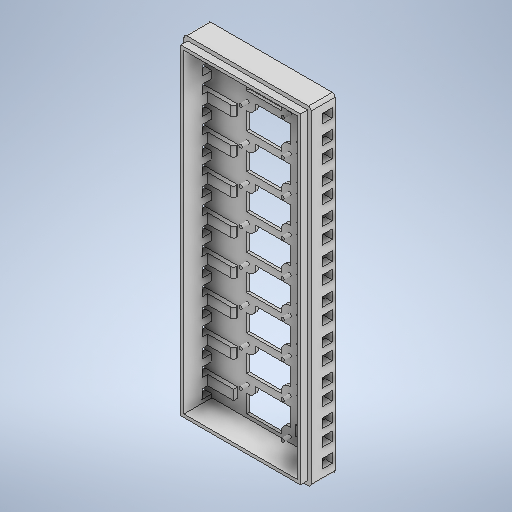
# Autodesk Inventor part: lm2596_socket_test
Saved by Autodesk Inventor 2025 (Build 290162000, 162)
## iProperties
Created: 2025-01-25
Part Number: lm2596_socket_test
Material: Všeobecné
Document SubType Name: Modeling
Designer: lukas
Density: 1 g/cm^3
Appearance: Výchozí
Author: lukas
## iProperties of the stored document lm2596_socket_3D tisk.ipt
Created: 2025-01-29
Part Number: lm2596_socket_3D tisk
Material: Všeobecné
Document SubType Name: Modeling
Designer: lukas
Density: 1 g/cm^3
Appearance: Výchozí
Author: lukas
Autodesk Inventor part; units mm, degrees
ref_plane "YZ Plane" through (0, 0, 0) normal (1, 0, 0) x (0, 1, 0)
ref_plane "XZ Plane" through (0, 0, 0) normal (0, 1, 0) x (-1, 0, 0)
sketch "Náčrt1" plane through (0, 0, 0) normal (0, 0, 1) x (1, 0, 0)
  line L0 (0, 17.5) -> (0, -17.5) projected
  line L1 (-32.9, 0) -> (32.9, 0) projected
  line L2 (23.5, -12.5) -> (-23.5, -12.5)
  line L3 (-23.5, -12.5) -> (-23.5, 12.5)
  line L4 (-23.5, 12.5) -> (23.5, 12.5)
  line L5 (23.5, 12.5) -> (23.5, -12.5)
  point P0 (0, 0)
  dimension "d0" = 47
  dimension "d1" = 25
  constraints: 8 end point, 2 parallel, 1 horizontal, 1 perpendicular, 2 other
  measures "d0" distance between parallel lines of L3 L5
  measures "d1" distance between parallel lines of L4 L2
extrude "Vysunutí1" add sketch "Náčrt1" along normal blind 2
sketch "Náčrt2" plane through (0, 0, 2) normal (0, 0, 1) x (1, 0, 0)
  line L0 (23.5, 12.5) -> (-23.5, 12.5) projected
  line L1 (-23.5, 12.5) -> (-23.5, -12.5) projected
  line L2 (-23.5, -12.5) -> (23.5, -12.5) projected
  line L3 (23.5, -12.5) -> (23.5, 12.5) projected
  line L4 (0, 17.5) -> (0, -17.5) projected
  line L5 (-32.9, 0) -> (32.9, 0) projected
  circle A0 centre (-15, 8.5) radius 1.2
  circle A1 centre (15, -8.5) radius 1.2
  point P0 (0, 0)
  dimension "d4" = 2.4
  dimension "d5" = 4
  dimension "d9" = 180
  dimension "d18" = 8.5
  constraints: 2 centre point, 3 other
  measures "d4" diameter of A0
  measures "d5" distance from line of A0.centre L0
  measures "d18" distance from line of L1 A0.centre
extrude "Vysunutí2" add sketch "Náčrt2" along normal blind 5 contours A0 | A1
sketch "Náčrt3" plane through (0, 0, 2) normal (0, 0, 1) x (1, 0, 0)
  circle A0 centre (15, -8.5) radius 1.2 projected
  circle A1 centre (-15, 8.5) radius 1.2 projected
  line L0 (23.5, 12.5) -> (-23.5, 12.5) projected
  line L1 (-23.5, 12.5) -> (-23.5, -12.5) projected
  line L2 (-23.5, -12.5) -> (23.5, -12.5) projected
  line L3 (23.5, -12.5) -> (23.5, 12.5) projected
  line L4 (0, 17.5) -> (0, -17.5) projected
  line L5 (-32.9, 0) -> (32.9, 0) projected
  line L6 (-23.5, 12.5) -> (-23.5, -12.5) projected
  line L7 (-22, -3.5) -> (-23.5, -3.5)
  line L8 (-23.5, -3.5) -> (-23.5, 3.5)
  line L9 (-23.5, 3.5) -> (-22, 3.5)
  line L10 (-22, 3.5) -> (-22, -3.5)
  line L11 (23.5, -3.5) -> (22, -3.5)
  line L12 (22, -3.5) -> (22, 3.5)
  line L13 (22, 3.5) -> (23.5, 3.5)
  line L14 (23.5, 3.5) -> (23.5, -3.5)
  line L15 (22, -3.5) -> (23.5, -3.5)
  line L16 (23.5, -3.5) -> (23.5, 0)
  line L17 (23.5, 0) -> (22, 0)
  line L18 (22, 0) -> (22, -3.5)
  line L19 (-22, -3.5) -> (-23.5, -3.5)
  line L20 (-23.5, -3.5) -> (-23.5, 0)
  line L21 (-23.5, 0) -> (-22, 0)
  line L22 (-22, 0) -> (-22, -3.5)
  point P0 (0, 0)
  point P1 (22, 0)
  point P2 (-22, 0)
  point P3 (-23.5, 3.5)
  point P4 (-23.5, -3.5)
  dimension "d13" = 7
  dimension "d14" = 7
  dimension "d15" = 44
  constraints: 32 end point, 8 parallel, 4 horizontal, 4 perpendicular, 2 midpoint, 2 point on line, 3 other
  measures "d13" distance of L9.end L7.start
  measures "d14" distance of L11.end L12.end
  measures "d15" distance between parallel lines of L10 L12
extrude "Vysunutí3" add sketch "Náčrt3" along normal blind 3 contours L3 L5 L12 L13 | L3 L11 L12 L5 | L9 L10 L5 L1 | L10 L7 L1 L5
sketch "Náčrt4" plane through (0, 0, 2) normal (0, 0, 1) x (1, 0, 0)
  line L0 (22, 3.5) -> (23.5, 3.5) projected
  line L1 (23.5, 3.5) -> (23.5, 12.5) projected
  line L2 (23.5, 12.5) -> (-23.5, 12.5) projected
  line L3 (-23.5, 12.5) -> (-23.5, 3.5) projected
  line L4 (-23.5, 3.5) -> (-22, 3.5) projected
  line L5 (-22, 3.5) -> (-22, -3.5) projected
  line L6 (-22, -3.5) -> (-23.5, -3.5) projected
  line L7 (-23.5, -3.5) -> (-23.5, -12.5) projected
  line L8 (-23.5, -12.5) -> (23.5, -12.5) projected
  line L9 (23.5, -12.5) -> (23.5, -3.5) projected
  line L10 (23.5, -3.5) -> (22, -3.5) projected
  line L11 (22, -3.5) -> (22, 3.5) projected
  circle A0 centre (15, -8.5) radius 1.2 projected
  circle A1 centre (-15, 8.5) radius 1.2 projected
  line L12 (15.8095, 10) -> (15.8095, -2.5549)
  line L13 (-15.8095, -10) -> (-15.8095, 2.5549)
  line L14 (0, 17.5) -> (0, -17.5) projected
  line L15 (-32.9, 0) -> (32.9, 0) projected
  arc A2 (-15.8095, 2.5549) -> (-9.1905, 10) centre (-15, 8.5) ccw
  arc A3 (15.8095, -2.5549) -> (9.1905, -10) centre (15, -8.5) ccw
  line L16 (-9.1905, 10) -> (15.8095, 10)
  line L17 (9.1905, -10) -> (-15.8095, -10)
  point P0 (0, 0)
  dimension "d21" = 12
  dimension "d22" = 12
  dimension "d23" = 20
  dimension "d25" = 25
  dimension "d26" = 25
  constraints: 8 end point, 4 point on circle, 2 centre point, 2 coincident, 2 parallel, 1 horizontal, 1 perpendicular, 1 other
  measures "d21" diameter of A2
  measures "d22" diameter of A3
  measures "d23" distance between parallel lines of L16 L17
  measures "d25" distance of L16.start L12.start
  measures "d26" distance of L17.start L13.start
extrude "Vysunutí4" cut sketch "Náčrt4" against normal through all contours L15 L14 L16 L12 | L12 A3 L17 L14 L15 | L15 L13 A2 L16 L14 | L14 L17 L13 L15
pattern_linear "Obdélníkové pole1" count 9 spacing 25 along (0, 1, 0) first direction both ways yes
sketch "Náčrt12" plane through (0, 0, 0) normal (0, 0, -1) x (-1, 0, 0)
  line L0 (15.8095, 15) -> (-9.1905, 15) projected
  arc A0 (-9.1905, 15) -> (-15.8095, 22.4451) centre (-15, 16.5) ccw projected
  line L1 (-15.8095, 22.4451) -> (-15.8095, 35) projected
  line L2 (-15.8095, 35) -> (9.1905, 35) projected
  arc A1 (9.1905, 35) -> (15.8095, 27.5549) centre (15, 33.5) ccw projected
  line L3 (15.8095, 27.5549) -> (15.8095, 15) projected
  line L4 (15.8095, 40) -> (-9.1905, 40) projected
  arc A2 (-9.1905, 40) -> (-15.8095, 47.4451) centre (-15, 41.5) ccw projected
  line L5 (-15.8095, 47.4451) -> (-15.8095, 60) projected
  line L6 (-15.8095, 60) -> (9.1905, 60) projected
  arc A3 (9.1905, 60) -> (15.8095, 52.5549) centre (15, 58.5) ccw projected
  line L7 (15.8095, 52.5549) -> (15.8095, 40) projected
  line L8 (15.8095, 65) -> (-9.1905, 65) projected
  arc A4 (-9.1905, 65) -> (-15.8095, 72.4451) centre (-15, 66.5) ccw projected
  line L9 (-15.8095, 72.4451) -> (-15.8095, 85) projected
  line L10 (-15.8095, 85) -> (9.1905, 85) projected
  arc A5 (9.1905, 85) -> (15.8095, 77.5549) centre (15, 83.5) ccw projected
  line L11 (15.8095, 77.5549) -> (15.8095, 65) projected
  line L12 (15.8095, 90) -> (-9.1905, 90) projected
  arc A6 (-9.1905, 90) -> (-15.8095, 97.4451) centre (-15, 91.5) ccw projected
  line L13 (-15.8095, 97.4451) -> (-15.8095, 110) projected
  line L14 (-15.8095, 110) -> (9.1905, 110) projected
  arc A7 (9.1905, 110) -> (15.8095, 102.5549) centre (15, 108.5) ccw projected
  line L15 (15.8095, 102.5549) -> (15.8095, 90) projected
  line L16 (15.8095, -110) -> (-9.1905, -110) projected
  arc A8 (-9.1905, -110) -> (-15.8095, -102.5549) centre (-15, -108.5) ccw projected
  line L17 (-15.8095, -102.5549) -> (-15.8095, -90) projected
  line L18 (-15.8095, -90) -> (9.1905, -90) projected
  arc A9 (9.1905, -90) -> (15.8095, -97.4451) centre (15, -91.5) ccw projected
  line L19 (15.8095, -97.4451) -> (15.8095, -110) projected
  line L20 (15.8095, -85) -> (-9.1905, -85) projected
  arc A10 (-9.1905, -85) -> (-15.8095, -77.5549) centre (-15, -83.5) ccw projected
  line L21 (-15.8095, -77.5549) -> (-15.8095, -65) projected
  line L22 (-15.8095, -65) -> (9.1905, -65) projected
  arc A11 (9.1905, -65) -> (15.8095, -72.4451) centre (15, -66.5) ccw projected
  line L23 (15.8095, -72.4451) -> (15.8095, -85) projected
  line L24 (15.8095, -60) -> (-9.1905, -60) projected
  arc A12 (-9.1905, -60) -> (-15.8095, -52.5549) centre (-15, -58.5) ccw projected
  line L25 (-15.8095, -52.5549) -> (-15.8095, -40) projected
  line L26 (-15.8095, -40) -> (9.1905, -40) projected
  arc A13 (9.1905, -40) -> (15.8095, -47.4451) centre (15, -41.5) ccw projected
  line L27 (15.8095, -47.4451) -> (15.8095, -60) projected
  line L28 (15.8095, -35) -> (-9.1905, -35) projected
  arc A14 (-9.1905, -35) -> (-15.8095, -27.5549) centre (-15, -33.5) ccw projected
  line L29 (-15.8095, -27.5549) -> (-15.8095, -15) projected
  line L30 (-15.8095, -15) -> (9.1905, -15) projected
  arc A15 (9.1905, -15) -> (15.8095, -22.4451) centre (15, -16.5) ccw projected
  line L31 (15.8095, -22.4451) -> (15.8095, -35) projected
  line L32 (15.8095, -10) -> (-9.1905, -10) projected
  arc A16 (-9.1905, -10) -> (-15.8095, -2.5549) centre (-15, -8.5) ccw projected
  line L33 (-15.8095, -2.5549) -> (-15.8095, 10) projected
  line L34 (-15.8095, 10) -> (9.1905, 10) projected
  arc A17 (9.1905, 10) -> (15.8095, 2.5549) centre (15, 8.5) ccw projected
  line L35 (15.8095, 2.5549) -> (15.8095, -10) projected
  line L36 (-23.5, -112.5) -> (-23.5, 112.5) projected
  line L37 (23.5, -112.5) -> (-23.5, -112.5) projected
  line L38 (23.5, 112.5) -> (23.5, -112.5) projected
  line L39 (-23.5, 112.5) -> (23.5, 112.5) projected
  line L40 (-45.5, 117.5) -> (45.5, 117.5)
  line L41 (45.5, 117.5) -> (45.5, -117.5)
  line L42 (45.5, -117.5) -> (-45.5, -117.5)
  line L43 (-45.5, -117.5) -> (-45.5, 117.5)
  line L44 (0, -164.5) -> (0, 164.5) projected
  line L45 (-63.7, 0) -> (63.7, 0) projected
  point P0 (0, 0)
  dimension "d53" = 22
  dimension "d54" = 5
  constraints: 8 end point, 2 parallel, 1 horizontal, 1 perpendicular, 2 other
  measures "d53" distance between parallel lines of L43 L36
  measures "d54" distance between parallel lines of L37 L42
extrude "Vysunutí12" add sketch "Náčrt12" against normal blind 2 contours L45 L43 L40 L44 L39 L36 | L36 L37 L44 L42 L43 L45 | L45 L41 L42 L44 L37 L38 | L38 L39 L44 L40 L41 L45
sketch "Náčrt13" plane through (0, 0, 2) normal (0, 0, 1) x (1, 0, 0)
  line L0 (-23.5, -21.5) -> (-22, -21.5) projected
  line L1 (-22, -21.5) -> (-22, -28.5) projected
  line L2 (-22, -28.5) -> (-23.5, -28.5) projected
  line L3 (-23.5, -21.5) -> (-23.5, -28.5) projected
  line L4 (-23.5, -46.5) -> (-22, -46.5) projected
  line L5 (-22, -46.5) -> (-22, -53.5) projected
  line L6 (-22, -53.5) -> (-23.5, -53.5) projected
  line L7 (-23.5, -46.5) -> (-23.5, -53.5) projected
  line L8 (-23.5, 3.5) -> (-23.5, -3.5) projected
  line L9 (-23.5, 3.5) -> (-22, 3.5) projected
  line L10 (-22, 3.5) -> (-22, -3.5) projected
  line L11 (-22, -3.5) -> (-23.5, -3.5) projected
  line L12 (-23.5, -71.5) -> (-22, -71.5) projected
  line L13 (-22, -71.5) -> (-22, -78.5) projected
  line L14 (-22, -78.5) -> (-23.5, -78.5) projected
  line L15 (-23.5, -71.5) -> (-23.5, -78.5) projected
  line L16 (23.5, -28.5) -> (22, -28.5) projected
  line L17 (22, -28.5) -> (22, -21.5) projected
  line L18 (22, -21.5) -> (23.5, -21.5) projected
  line L19 (23.5, -28.5) -> (23.5, -21.5) projected
  line L20 (23.5, -53.5) -> (23.5, -46.5) projected
  line L21 (23.5, -53.5) -> (22, -53.5) projected
  line L22 (22, -53.5) -> (22, -46.5) projected
  line L23 (22, -46.5) -> (23.5, -46.5) projected
  line L24 (-23.5, 28.5) -> (-23.5, 21.5) projected
  line L25 (-23.5, 28.5) -> (-22, 28.5) projected
  line L26 (-22, 28.5) -> (-22, 21.5) projected
  line L27 (-22, 21.5) -> (-23.5, 21.5) projected
  line L28 (-23.5, -96.5) -> (-22, -96.5) projected
  line L29 (-22, -96.5) -> (-22, -103.5) projected
  line L30 (-22, -103.5) -> (-23.5, -103.5) projected
  line L31 (-23.5, -96.5) -> (-23.5, -103.5) projected
  line L32 (23.5, -3.5) -> (22, -3.5) projected
  line L33 (22, -3.5) -> (22, 3.5) projected
  line L34 (22, 3.5) -> (23.5, 3.5) projected
  line L35 (23.5, -3.5) -> (23.5, 3.5) projected
  line L36 (23.5, -78.5) -> (23.5, -71.5) projected
  line L37 (23.5, -78.5) -> (22, -78.5) projected
  line L38 (22, -78.5) -> (22, -71.5) projected
  line L39 (22, -71.5) -> (23.5, -71.5) projected
  line L40 (-23.5, 53.5) -> (-23.5, 46.5) projected
  line L41 (-23.5, 53.5) -> (-22, 53.5) projected
  line L42 (-22, 53.5) -> (-22, 46.5) projected
  line L43 (-22, 46.5) -> (-23.5, 46.5) projected
  line L44 (23.5, 21.5) -> (22, 21.5) projected
  line L45 (22, 21.5) -> (22, 28.5) projected
  line L46 (22, 28.5) -> (23.5, 28.5) projected
  line L47 (23.5, 21.5) -> (23.5, 28.5) projected
  line L48 (23.5, -103.5) -> (23.5, -96.5) projected
  line L49 (23.5, -103.5) -> (22, -103.5) projected
  line L50 (22, -103.5) -> (22, -96.5) projected
  line L51 (22, -96.5) -> (23.5, -96.5) projected
  line L52 (-23.5, 78.5) -> (-23.5, 71.5) projected
  line L53 (-23.5, 78.5) -> (-22, 78.5) projected
  line L54 (-22, 78.5) -> (-22, 71.5) projected
  line L55 (-22, 71.5) -> (-23.5, 71.5) projected
  line L56 (23.5, 46.5) -> (22, 46.5) projected
  line L57 (22, 46.5) -> (22, 53.5) projected
  line L58 (22, 53.5) -> (23.5, 53.5) projected
  line L59 (23.5, 46.5) -> (23.5, 53.5) projected
  line L60 (23.5, 71.5) -> (22, 71.5) projected
  line L61 (22, 71.5) -> (22, 78.5) projected
  line L62 (22, 78.5) -> (23.5, 78.5) projected
  line L63 (23.5, 71.5) -> (23.5, 78.5) projected
  line L64 (-23.5, 103.5) -> (-23.5, 96.5) projected
  line L65 (-23.5, 103.5) -> (-22, 103.5) projected
  line L66 (-22, 103.5) -> (-22, 96.5) projected
  line L67 (-22, 96.5) -> (-23.5, 96.5) projected
  line L68 (45.5, -117.5) -> (45.5, 117.5) projected
  line L69 (45.5, 117.5) -> (-45.5, 117.5) projected
  line L70 (-45.5, 117.5) -> (-45.5, -117.5) projected
  line L71 (-45.5, -117.5) -> (45.5, -117.5) projected
  circle A0 centre (-15, 33.5) radius 1.2 projected
  circle A1 centre (15, 16.5) radius 1.2 projected
  line L72 (9.1905, 15) -> (-15.8095, 15) projected
  line L73 (-15.8095, 15) -> (-15.8095, 27.5549) projected
  arc A2 (-15.8095, 27.5549) -> (-9.1905, 35) centre (-15, 33.5) ccw projected
  line L74 (-9.1905, 35) -> (15.8095, 35) projected
  line L75 (15.8095, 35) -> (15.8095, 22.4451) projected
  arc A3 (15.8095, 22.4451) -> (9.1905, 15) centre (15, 16.5) ccw projected
  line L76 (9.1905, 40) -> (-15.8095, 40) projected
  line L77 (-15.8095, 40) -> (-15.8095, 52.5549) projected
  arc A4 (-15.8095, 52.5549) -> (-9.1905, 60) centre (-15, 58.5) ccw projected
  line L78 (-9.1905, 60) -> (15.8095, 60) projected
  line L79 (15.8095, 60) -> (15.8095, 47.4451) projected
  arc A5 (15.8095, 47.4451) -> (9.1905, 40) centre (15, 41.5) ccw projected
  circle A6 centre (15, 41.5) radius 1.2 projected
  circle A7 centre (-15, 58.5) radius 1.2 projected
  line L80 (9.1905, 65) -> (-15.8095, 65) projected
  line L81 (-15.8095, 65) -> (-15.8095, 77.5549) projected
  arc A8 (-15.8095, 77.5549) -> (-9.1905, 85) centre (-15, 83.5) ccw projected
  line L82 (-9.1905, 85) -> (15.8095, 85) projected
  line L83 (15.8095, 85) -> (15.8095, 72.4451) projected
  arc A9 (15.8095, 72.4451) -> (9.1905, 65) centre (15, 66.5) ccw projected
  circle A10 centre (15, 66.5) radius 1.2 projected
  circle A11 centre (-15, 83.5) radius 1.2 projected
  line L84 (9.1905, 90) -> (-15.8095, 90) projected
  line L85 (-15.8095, 90) -> (-15.8095, 102.5549) projected
  arc A12 (-15.8095, 102.5549) -> (-9.1905, 110) centre (-15, 108.5) ccw projected
  line L86 (-9.1905, 110) -> (15.8095, 110) projected
  line L87 (15.8095, 110) -> (15.8095, 97.4451) projected
  arc A13 (15.8095, 97.4451) -> (9.1905, 90) centre (15, 91.5) ccw projected
  circle A14 centre (15, 91.5) radius 1.2 projected
  circle A15 centre (-15, 108.5) radius 1.2 projected
  circle A16 centre (-15, -91.5) radius 1.2 projected
  circle A17 centre (15, -108.5) radius 1.2 projected
  line L88 (9.1905, -110) -> (-15.8095, -110) projected
  line L89 (-15.8095, -110) -> (-15.8095, -97.4451) projected
  arc A18 (-15.8095, -97.4451) -> (-9.1905, -90) centre (-15, -91.5) ccw projected
  line L90 (-9.1905, -90) -> (15.8095, -90) projected
  line L91 (15.8095, -90) -> (15.8095, -102.5549) projected
  arc A19 (15.8095, -102.5549) -> (9.1905, -110) centre (15, -108.5) ccw projected
  line L92 (9.1905, -85) -> (-15.8095, -85) projected
  line L93 (-15.8095, -85) -> (-15.8095, -72.4451) projected
  arc A20 (-15.8095, -72.4451) -> (-9.1905, -65) centre (-15, -66.5) ccw projected
  line L94 (-9.1905, -65) -> (15.8095, -65) projected
  line L95 (15.8095, -65) -> (15.8095, -77.5549) projected
  arc A21 (15.8095, -77.5549) -> (9.1905, -85) centre (15, -83.5) ccw projected
  circle A22 centre (15, -83.5) radius 1.2 projected
  circle A23 centre (-15, -66.5) radius 1.2 projected
  line L96 (9.1905, -60) -> (-15.8095, -60) projected
  line L97 (-15.8095, -60) -> (-15.8095, -47.4451) projected
  arc A24 (-15.8095, -47.4451) -> (-9.1905, -40) centre (-15, -41.5) ccw projected
  line L98 (-9.1905, -40) -> (15.8095, -40) projected
  line L99 (15.8095, -40) -> (15.8095, -52.5549) projected
  arc A25 (15.8095, -52.5549) -> (9.1905, -60) centre (15, -58.5) ccw projected
  circle A26 centre (15, -58.5) radius 1.2 projected
  circle A27 centre (-15, -41.5) radius 1.2 projected
  line L100 (9.1905, -35) -> (-15.8095, -35) projected
  line L101 (-15.8095, -35) -> (-15.8095, -22.4451) projected
  arc A28 (-15.8095, -22.4451) -> (-9.1905, -15) centre (-15, -16.5) ccw projected
  line L102 (-9.1905, -15) -> (15.8095, -15) projected
  line L103 (15.8095, -15) -> (15.8095, -27.5549) projected
  arc A29 (15.8095, -27.5549) -> (9.1905, -35) centre (15, -33.5) ccw projected
  circle A30 centre (15, -33.5) radius 1.2 projected
  circle A31 centre (-15, -16.5) radius 1.2 projected
  line L104 (9.1905, -10) -> (-15.8095, -10) projected
  line L105 (-15.8095, -10) -> (-15.8095, 2.5549) projected
  arc A32 (-15.8095, 2.5549) -> (-9.1905, 10) centre (-15, 8.5) ccw projected
  line L106 (-9.1905, 10) -> (15.8095, 10) projected
  line L107 (15.8095, 10) -> (15.8095, -2.5549) projected
  arc A33 (15.8095, -2.5549) -> (9.1905, -10) centre (15, -8.5) ccw projected
  line L108 (23.5, 96.5) -> (23.5, 103.5) projected
  line L109 (23.5, 96.5) -> (22, 96.5) projected
  line L110 (22, 96.5) -> (22, 103.5) projected
  line L111 (22, 103.5) -> (23.5, 103.5) projected
  circle A34 centre (15, -8.5) radius 1.2 projected
  circle A35 centre (-15, 8.5) radius 1.2 projected
  line L112 (0, 164.5) -> (0, -164.5) projected
  line L113 (-63.7, 0) -> (63.7, 0) projected
  line L114 (45.5, -117.5) -> (45.5, 117.5) projected
  line L115 (45.5, 117.5) -> (-45.5, 117.5)
  line L116 (-45.5, 117.5) -> (-45.5, -117.5)
  line L117 (-45.5, -117.5) -> (45.5, -117.5)
  line L118 (45.5, -117.5) -> (45.5, 117.5)
  line L119 (40.5, 112.5) -> (-40.5, 112.5)
  line L120 (-40.5, 112.5) -> (-40.5, -112.5)
  line L121 (-40.5, -112.5) -> (40.5, -112.5)
  line L122 (40.5, -112.5) -> (40.5, 112.5)
  line L123 (45.5, 117.5) -> (-45.5, 117.5)
  line L124 (-45.5, 117.5) -> (-45.5, -117.5)
  line L125 (-45.5, -117.5) -> (45.5, -117.5)
  line L126 (45.5, -117.5) -> (45.5, 117.5)
  line L127 (45.5, 0) -> (40.5, 0)
  line L128 (40.5, -112.5) -> (0, -112.5)
  line L129 (-40.5, -112.5) -> (-40.5, 0)
  line L130 (-45.5, 117.5) -> (-45.5, -117.5) projected
  line L131 (-45.5, 0) -> (-45.5, -117.5)
  line L132 (-45.5, -117.5) -> (45.5, -117.5)
  line L133 (45.5, 0) -> (45.5, -117.5)
  line L134 (40.5, 0) -> (40.5, -112.5)
  line L135 (0, -112.5) -> (40.5, -112.5)
  line L136 (-45.5, -117.5) -> (45.5, -117.5) projected
  line L137 (0, -117.5) -> (0, -112.5)
  line L138 (0, -117.5) -> (45.5, -117.5)
  line L139 (45.5, -117.5) -> (45.5, 0)
  line L140 (45.5, 0) -> (40.5, 0)
  point P0 (0, 0)
  dimension "d59" = 5
  constraints: 48 end point, 6 midpoint, 6 parallel, 6 perpendicular, 5 collinear, 2 horizontal, 1 vertical, 3 other
  measures "d59" distance between parallel lines of L118 L122
extrude "Vysunutí13" add sketch "Náčrt13" along normal blind 15 contours L120 L121 L112 L71 L70 L113 | L113 L70 L69 L112 L119 L120 | L112 L69 L68 L113 L122 L119 | L121 L122 L113 L68 L71 L112
sketch "Náčrt14" plane through (-45.5, -117.5, 0) normal (-1, 0, 0) x (0, 0, 1)
  line L0 (-3.4, 117.5) -> (20.4, 117.5) projected
  line L1 (0, 282) -> (0, -47) projected
  line L2 (2, 230) -> (17, 230) projected
  line L3 (2, 230) -> (17, 230) projected
  line L4 (2, 221) -> (2, 214) projected
  line L5 (2, 214) -> (5, 214) projected
  line L6 (5, 221) -> (5, 214) projected
  line L7 (2, 221) -> (5, 221) projected
  line L8 (2, 5) -> (2, 230) projected
  line L9 (2, 230) -> (2, 5) projected
  line L10 (2, 96) -> (2, 89) projected
  line L11 (2, 96) -> (2, 89) projected
  line L12 (2, 71) -> (2, 64) projected
  line L13 (2, 71) -> (2, 64) projected
  line L14 (2, 121) -> (2, 114) projected
  line L15 (2, 121) -> (2, 114) projected
  line L16 (2, 46) -> (2, 39) projected
  line L17 (2, 46) -> (2, 39) projected
  line L18 (2, 89) -> (2, 96) projected
  line L19 (2, 89) -> (2, 96) projected
  line L20 (2, 64) -> (2, 71) projected
  line L21 (2, 64) -> (2, 71) projected
  line L22 (2, 146) -> (2, 139) projected
  line L23 (2, 146) -> (2, 139) projected
  line L24 (2, 21) -> (2, 14) projected
  line L25 (2, 21) -> (2, 14) projected
  line L26 (2, 114) -> (2, 121) projected
  line L27 (2, 114) -> (2, 121) projected
  line L28 (2, 39) -> (2, 46) projected
  line L29 (2, 39) -> (2, 46) projected
  line L30 (2, 171) -> (2, 164) projected
  line L31 (2, 171) -> (2, 164) projected
  line L32 (2, 139) -> (2, 146) projected
  line L33 (2, 139) -> (2, 146) projected
  line L34 (2, 14) -> (2, 21) projected
  line L35 (2, 14) -> (2, 21) projected
  line L36 (2, 196) -> (2, 189) projected
  line L37 (2, 196) -> (2, 189) projected
  line L38 (2, 164) -> (2, 171) projected
  line L39 (2, 164) -> (2, 171) projected
  line L40 (2, 189) -> (2, 196) projected
  line L41 (2, 189) -> (2, 196) projected
  line L42 (2, 221) -> (2, 214) projected
  line L43 (2, 221) -> (2, 214) projected
  line L44 (2, 152.2) -> (2, 149.8) projected
  line L45 (2, 135.2) -> (2, 132.8) projected
  line L46 (2, 132.5) -> (2, 145.0549) projected
  line L47 (2, 145.0549) -> (2, 152.5) projected
  line L48 (2, 152.5) -> (2, 139.9451) projected
  line L49 (2, 139.9451) -> (2, 132.5) projected
  line L50 (2, 157.5) -> (2, 170.0549) projected
  line L51 (2, 170.0549) -> (2, 177.5) projected
  line L52 (2, 177.5) -> (2, 164.9451) projected
  line L53 (2, 164.9451) -> (2, 157.5) projected
  line L54 (2, 160.2) -> (2, 157.8) projected
  line L55 (2, 177.2) -> (2, 174.8) projected
  line L56 (2, 182.5) -> (2, 195.0549) projected
  line L57 (2, 195.0549) -> (2, 202.5) projected
  line L58 (2, 202.5) -> (2, 189.9451) projected
  line L59 (2, 189.9451) -> (2, 182.5) projected
  line L60 (2, 185.2) -> (2, 182.8) projected
  line L61 (2, 202.2) -> (2, 199.8) projected
  line L62 (2, 207.5) -> (2, 220.0549) projected
  line L63 (2, 220.0549) -> (2, 227.5) projected
  line L64 (2, 227.5) -> (2, 214.9451) projected
  line L65 (2, 214.9451) -> (2, 207.5) projected
  line L66 (2, 210.2) -> (2, 207.8) projected
  line L67 (2, 227.2) -> (2, 224.8) projected
  line L68 (2, 27.2) -> (2, 24.8) projected
  line L69 (2, 10.2) -> (2, 7.8) projected
  line L70 (2, 7.5) -> (2, 20.0549) projected
  line L71 (2, 20.0549) -> (2, 27.5) projected
  line L72 (2, 27.5) -> (2, 14.9451) projected
  line L73 (2, 14.9451) -> (2, 7.5) projected
  line L74 (2, 32.5) -> (2, 45.0549) projected
  line L75 (2, 45.0549) -> (2, 52.5) projected
  line L76 (2, 52.5) -> (2, 39.9451) projected
  line L77 (2, 39.9451) -> (2, 32.5) projected
  line L78 (2, 35.2) -> (2, 32.8) projected
  line L79 (2, 52.2) -> (2, 49.8) projected
  line L80 (2, 57.5) -> (2, 70.0549) projected
  line L81 (2, 70.0549) -> (2, 77.5) projected
  line L82 (2, 77.5) -> (2, 64.9451) projected
  line L83 (2, 64.9451) -> (2, 57.5) projected
  line L84 (2, 60.2) -> (2, 57.8) projected
  line L85 (2, 77.2) -> (2, 74.8) projected
  line L86 (2, 82.5) -> (2, 95.0549) projected
  line L87 (2, 95.0549) -> (2, 102.5) projected
  line L88 (2, 102.5) -> (2, 89.9451) projected
  line L89 (2, 89.9451) -> (2, 82.5) projected
  line L90 (2, 85.2) -> (2, 82.8) projected
  line L91 (2, 102.2) -> (2, 99.8) projected
  line L92 (2, 107.5) -> (2, 120.0549) projected
  line L93 (2, 120.0549) -> (2, 127.5) projected
  line L94 (2, 127.5) -> (2, 114.9451) projected
  line L95 (2, 114.9451) -> (2, 107.5) projected
  line L96 (2, 214) -> (2, 221) projected
  line L97 (2, 214) -> (2, 221) projected
  line L98 (2, 110.2) -> (2, 107.8) projected
  line L99 (2, 127.2) -> (2, 124.8) projected
  line L100 (2, 5) -> (17, 5) projected
  line L101 (2, 230) -> (9, 230)
  line L102 (9, 230) -> (9, 5)
  line L103 (9, 5) -> (2, 5)
  line L104 (2, 5) -> (2, 230)
  line L105 (2, 196) -> (2, 189) projected
  line L106 (2, 189) -> (5, 189) projected
  line L107 (5, 196) -> (5, 189) projected
  line L108 (2, 196) -> (5, 196) projected
  line L109 (2, 171) -> (2, 164) projected
  line L110 (2, 164) -> (5, 164) projected
  line L111 (5, 171) -> (5, 164) projected
  line L112 (2, 171) -> (5, 171) projected
  line L113 (2, 146) -> (2, 139) projected
  line L114 (2, 139) -> (5, 139) projected
  line L115 (5, 146) -> (5, 139) projected
  line L116 (2, 146) -> (5, 146) projected
  line L117 (2, 121) -> (2, 114) projected
  line L118 (2, 114) -> (5, 114) projected
  line L119 (5, 121) -> (5, 114) projected
  line L120 (2, 121) -> (5, 121) projected
  line L121 (2, 96) -> (2, 89) projected
  line L122 (2, 89) -> (5, 89) projected
  line L123 (5, 96) -> (5, 89) projected
  line L124 (2, 96) -> (5, 96) projected
  line L125 (2, 71) -> (2, 64) projected
  line L126 (2, 64) -> (5, 64) projected
  line L127 (5, 71) -> (5, 64) projected
  line L128 (2, 71) -> (5, 71) projected
  line L129 (2, 46) -> (2, 39) projected
  line L130 (2, 39) -> (5, 39) projected
  line L131 (5, 46) -> (5, 39) projected
  line L132 (2, 46) -> (5, 46) projected
  line L133 (2, 21) -> (2, 14) projected
  line L134 (2, 14) -> (5, 14) projected
  line L135 (5, 21) -> (5, 14) projected
  line L136 (2, 21) -> (5, 21) projected
  line L137 (2, 221) -> (9, 221)
  line L138 (9, 221) -> (9, 214)
  line L139 (9, 214) -> (2, 214)
  line L140 (2, 214) -> (2, 221)
  line L141 (2, 196) -> (9, 196)
  line L142 (9, 196) -> (9, 189)
  line L143 (9, 189) -> (2, 189)
  line L144 (2, 189) -> (2, 196)
  line L145 (2, 171) -> (9, 171)
  line L146 (9, 171) -> (9, 164)
  line L147 (9, 164) -> (2, 164)
  line L148 (2, 164) -> (2, 171)
  line L149 (2, 146) -> (9, 146)
  line L150 (9, 146) -> (9, 139)
  line L151 (9, 139) -> (2, 139)
  line L152 (2, 139) -> (2, 146)
  line L153 (2, 121) -> (9, 121)
  line L154 (9, 121) -> (9, 114)
  line L155 (9, 114) -> (2, 114)
  line L156 (2, 114) -> (2, 121)
  line L157 (2, 96) -> (9, 96)
  line L158 (9, 96) -> (9, 89)
  line L159 (9, 89) -> (2, 89)
  line L160 (2, 89) -> (2, 96)
  line L161 (2, 71) -> (9, 71)
  line L162 (9, 71) -> (9, 64)
  line L163 (9, 64) -> (2, 64)
  line L164 (2, 64) -> (2, 71)
  line L165 (2, 46) -> (9, 46)
  line L166 (9, 46) -> (9, 39)
  line L167 (9, 39) -> (2, 39)
  line L168 (2, 39) -> (2, 46)
  line L169 (2, 21) -> (9, 21)
  line L170 (9, 21) -> (9, 14)
  line L171 (9, 14) -> (2, 14)
  line L172 (2, 14) -> (2, 21)
  line L173 (2, 207.5) -> (0, 207.5) projected
  line L174 (2, 202.5) -> (0, 202.5) projected
  line L175 (2, 207.5) -> (9, 207.5)
  line L176 (2, 202.5) -> (9, 202.5)
  line L177 (2, 182.5) -> (0, 182.5) projected
  line L178 (2, 177.5) -> (0, 177.5) projected
  line L179 (2, 152.5) -> (0, 152.5) projected
  line L180 (2, 127.5) -> (0, 127.5) projected
  line L181 (2, 102.5) -> (0, 102.5) projected
  line L182 (2, 77.5) -> (0, 77.5) projected
  line L183 (2, 52.5) -> (0, 52.5) projected
  line L184 (2, 27.5) -> (0, 27.5) projected
  line L185 (2, 32.5) -> (0, 32.5) projected
  line L186 (2, 57.5) -> (0, 57.5) projected
  line L187 (2, 82.5) -> (0, 82.5) projected
  line L188 (2, 107.5) -> (0, 107.5) projected
  line L189 (2, 132.5) -> (0, 132.5) projected
  line L190 (2, 157.5) -> (0, 157.5) projected
  line L191 (2, 182.5) -> (9, 182.5)
  line L192 (2, 177.5) -> (9, 177.5)
  line L193 (2, 157.5) -> (9, 157.5)
  line L194 (2, 152.5) -> (9, 152.5)
  line L195 (2, 132.5) -> (9, 132.5)
  line L196 (2, 127.5) -> (9, 127.5)
  line L197 (2, 107.5) -> (9, 107.5)
  line L198 (2, 102.5) -> (9, 102.5)
  line L199 (2, 82.5) -> (9, 82.5)
  line L200 (2, 77.5) -> (9, 77.5)
  line L201 (2, 57.5) -> (9, 57.5)
  line L202 (2, 52.5) -> (9, 52.5)
  line L203 (2, 32.5) -> (9, 32.5)
  line L204 (2, 27.5) -> (9, 27.5)
  line L205 (2, 227.5) -> (0, 227.5) projected
  line L206 (2, 7.5) -> (0, 7.5) projected
  line L207 (2, 227.5) -> (9, 227.5)
  line L208 (2, 7.5) -> (9, 7.5)
  point P0 (0, 117.5)
  point P1 (9, 21)
  point P2 (9, 71)
  point P3 (9, 46)
  point P4 (9, 96)
  point P5 (9, 146)
  point P6 (9, 221)
  point P7 (9, 230)
  point P8 (2, 230)
  dimension "d62" = 7
  constraints: 114 end point, 27 horizontal, 20 parallel, 11 point on line, 9 perpendicular, 1 vertical, 32 other
extrude "Vysunutí14" cut sketch "Náčrt14" against normal up to surface (5 mm away) contours L196 L102 L153 L120 L8 | L8 L118 L155 L102 L197 | L8 L114 L151 L102 L195 | L198 L102 L157 L124 L8 | L194 L102 L149 L116 L8 | L8 L122 L159 L102 L199 | L8 L110 L147 L102 L193 | L200 L102 L161 L128 L8 | L192 L102 L145 L112 L8 | L8 L126 L163 L102 L201 | L8 L106 L143 L102 L191 | L202 L102 L165 L132 L8 | L176 L102 L141 L108 L8 | L8 L130 L167 L102 L203 | L8 L5 L139 L102 L175 | L204 L102 L169 L136 L8 | L207 L102 L137 L7 L8 | L8 L134 L171 L102 L208
sketch "Náčrt15" plane through (-23.5, 96.5, 2) normal (-1, 0, 0) x (0, 0, 1)
  line L0 (0, 7) -> (0, 0) projected
  line L1 (0, 0) -> (3, 0) projected
  line L2 (3, 7) -> (3, 0) projected
  line L3 (0, 7) -> (3, 7) projected
  line L4 (3, 7) -> (3, 0) projected
  line L5 (0, 0) -> (3, 0)
  line L6 (3, 0) -> (3, 7)
  line L7 (3, 7) -> (0, 7)
  line L8 (0, 7) -> (0, 0)
  line L9 (0, -18) -> (0, -25) projected
  line L10 (0, -18) -> (0, -25) projected
  line L11 (0, -25) -> (3, -25) projected
  line L12 (3, -18) -> (3, -25) projected
  line L13 (0, -18) -> (3, -18) projected
  line L14 (0, -43) -> (0, -50) projected
  line L15 (0, -50) -> (3, -50) projected
  line L16 (3, -43) -> (3, -50) projected
  line L17 (0, -43) -> (3, -43) projected
  line L18 (0, -68) -> (0, -75) projected
  line L19 (0, -75) -> (3, -75) projected
  line L20 (3, -68) -> (3, -75) projected
  line L21 (0, -68) -> (3, -68) projected
  line L22 (0, -93) -> (0, -100) projected
  line L23 (0, -100) -> (3, -100) projected
  line L24 (3, -93) -> (3, -100) projected
  line L25 (0, -93) -> (3, -93) projected
  line L26 (0, -118) -> (0, -125) projected
  line L27 (0, -125) -> (3, -125) projected
  line L28 (3, -118) -> (3, -125) projected
  line L29 (0, -118) -> (3, -118) projected
  line L30 (0, -143) -> (0, -150) projected
  line L31 (0, -150) -> (3, -150) projected
  line L32 (3, -143) -> (3, -150) projected
  line L33 (0, -143) -> (3, -143) projected
  line L34 (0, -168) -> (0, -175) projected
  line L35 (0, -175) -> (3, -175) projected
  line L36 (3, -168) -> (3, -175) projected
  line L37 (0, -168) -> (3, -168) projected
  line L38 (0, -193) -> (0, -200) projected
  line L39 (0, -200) -> (3, -200) projected
  line L40 (3, -193) -> (3, -200) projected
  line L41 (0, -193) -> (3, -193) projected
  line L42 (0, -193) -> (0, -200) projected
  line L43 (3, -193) -> (3, -200) projected
  line L44 (0, -200) -> (3, -200)
  line L45 (3, -200) -> (3, -193)
  line L46 (3, -193) -> (0, -193)
  line L47 (0, -193) -> (0, -200)
  line L48 (0, -168) -> (0, -175) projected
  line L49 (0, -175) -> (3, -175)
  line L50 (3, -175) -> (3, -168)
  line L51 (3, -168) -> (0, -168)
  line L52 (0, -168) -> (0, -175)
  line L53 (0, -150) -> (3, -150) projected
  line L54 (0, -150) -> (3, -150)
  line L55 (3, -150) -> (3, -143)
  line L56 (3, -143) -> (0, -143)
  line L57 (0, -143) -> (0, -150)
  line L58 (0, -118) -> (0, -125) projected
  line L59 (0, -125) -> (3, -125)
  line L60 (3, -125) -> (3, -118)
  line L61 (3, -118) -> (0, -118)
  line L62 (0, -118) -> (0, -125)
  line L63 (0, -93) -> (0, -100) projected
  line L64 (0, -100) -> (3, -100)
  line L65 (3, -100) -> (3, -93)
  line L66 (3, -93) -> (0, -93)
  line L67 (0, -93) -> (0, -100)
  line L68 (0, -68) -> (0, -75) projected
  line L69 (0, -75) -> (3, -75)
  line L70 (3, -75) -> (3, -68)
  line L71 (3, -68) -> (0, -68)
  line L72 (0, -68) -> (0, -75)
  line L73 (3, -43) -> (3, -50) projected
  line L74 (0, -50) -> (3, -50)
  line L75 (3, -50) -> (3, -43)
  line L76 (3, -43) -> (0, -43)
  line L77 (0, -43) -> (0, -50)
  line L78 (0, -18) -> (0, -25) projected
  line L79 (0, -25) -> (3, -25)
  line L80 (3, -25) -> (3, -18)
  line L81 (3, -18) -> (0, -18)
  line L82 (0, -18) -> (0, -25)
  point P0 (-2, -96.5)
  constraints: 72 end point, 18 parallel, 9 horizontal, 9 perpendicular
extrude "Vysunutí15" add sketch "Náčrt15" along normal up to surface (17 mm away)
fillet "Zaoblení5" radius 2 4 edges at (-45.5, 117.5, 8.5) (-45.5, -117.5, 8.5) (45.5, -117.5, 8.5) (45.5, 117.5, 8.5)
ref_plane "Pracovní rovina1" through (0, -115.5, 0) normal (-1, 0, 0) x (0, 0, 1)
mirror "Zrcadlit2" about plane through (0, -115.5, 0) normal (-1, 0, 0) of "Vysunutí14"
mirror "Zrcadlit3" about plane through (0, -115.5, 0) normal (-1, 0, 0) of "Vysunutí15"
fillet "Zaoblení6" radius 2 16 edges at (-22, 100, 5) (-22, 75, 5) (-22, 50, 5) (-22, 25, 5) (-22, 0, 5) (-22, -25, 5) (-22, -50, 5) (-22, -75, 5) (22, -75, 5) (22, -50, 5) (22, -25, 5) (22, 0, 5) (22, 25, 5) (22, 50, 5) (22, 75, 5) (22, 100, 5)
sketch "Náčrt16" plane through (0, 0, 17) normal (0, 0, 1) x (1, 0, 0)
  arc A0 (45.5, 115.5) -> (43.5, 117.5) centre (43.5, 115.5) ccw projected
  line L0 (43.5, 117.5) -> (-43.5, 117.5) projected
  arc A1 (-43.5, 117.5) -> (-45.5, 115.5) centre (-43.5, 115.5) ccw projected
  line L1 (-45.5, 115.5) -> (-45.5, -115.5) projected
  arc A2 (-45.5, -115.5) -> (-43.5, -117.5) centre (-43.5, -115.5) ccw projected
  line L2 (-43.5, -117.5) -> (43.5, -117.5) projected
  arc A3 (43.5, -117.5) -> (45.5, -115.5) centre (43.5, -115.5) ccw projected
  line L3 (45.5, -115.5) -> (45.5, 115.5) projected
  line L4 (-40.5, -112.5) -> (-40.5, 112.5) projected
  line L5 (-40.5, 112.5) -> (40.5, 112.5) projected
  line L6 (40.5, 112.5) -> (40.5, -112.5) projected
  line L7 (40.5, -112.5) -> (-40.5, -112.5) projected
  line L8 (0, 165.0799) -> (0, -165.0799) projected
  line L9 (-64.2799, 0) -> (64.2799, 0) projected
  line L10 (-45.5, -112.5) -> (-40.5, -112.5) projected
  line L11 (40.5, 112.5) -> (-40.5, 112.5)
  line L12 (-40.5, 112.5) -> (-40.5, -112.5)
  line L13 (-40.5, -112.5) -> (40.5, -112.5)
  line L14 (40.5, -112.5) -> (40.5, 112.5)
  line L15 (42.75, 114.75) -> (-42.75, 114.75)
  line L16 (-42.75, 114.75) -> (-42.75, -114.75)
  line L17 (-42.75, -114.75) -> (42.75, -114.75)
  line L18 (42.75, -114.75) -> (42.75, 114.75)
  point P0 (0, 0)
  dimension "d69" = 2.25
  constraints: 16 end point, 4 parallel, 2 perpendicular, 1 horizontal, 3 other
  measures "d69" distance between parallel lines of L14 L18
extrude "Vysunutí16" add sketch "Náčrt16" along normal blind 5 contours L18 L17 L8 L7 L6 L9 | L9 L6 L5 L8 L15 L18 | L8 L5 L4 L9 L16 L15 | L17 L16 L10 L7 L8 | L9 L4 L10 L16
